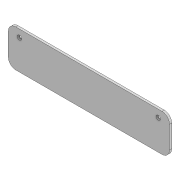
# Autodesk Inventor part: rackback
Saved by Autodesk Inventor 2020 (Build 240168000, 168)
## iProperties
Created: 2021-06-15
Part Number: rackback
Material: Generic
Document SubType Name: Modeling
Designer: Aidan Lee
Density: 1 g/cm^3
Appearance: Default
Author: Aidan Lee
Autodesk Inventor part; units mm, degrees
ref_plane "YZ Plane" through (0, 0, 0) normal (1, 0, 0) x (0, 1, 0)
ref_plane "XZ Plane" through (0, 0, 0) normal (0, 1, 0) x (-1, 0, 0)
ref_plane "XY Plane" through (0, 0, 0) normal (0, 0, 1) x (1, 0, 0)
sketch "Sketch1" plane through (0, 0, 0) normal (0, 0, 1) x (1, 0, 0)
  line L0 (0, 0) -> (215.985, 0)
  line L1 (215.985, 0) -> (215.985, 50)
  line L2 (215.985, 50) -> (0, 50)
  line L3 (0, 50) -> (0, 0)
  circle A0 centre (15, 40) radius 3
  line L4 (107.9925, 95.9564) -> (107.9925, 80.5337) construction
  circle A1 centre (200.985, 40) radius 3
  point P0 (107.9925, 50)
  point P1 (107.9925, 88.2451)
  dimension "d0" = 50
  dimension "d1" = 215.985
  dimension "d2" = 6
  dimension "d3" = 15
  dimension "d4" = 10
  constraints: 10 end point, 2 centre point, 2 midpoint, 2 parallel, 1 horizontal, 1 perpendicular, 1 symmetric about line, 1 vertical, 1 vertical alignment, 1 other
  measures "d0" distance of L2.end L0.start
  measures "d1" distance of L0.start L0.end
  measures "d2" diameter of A0
  measures "d3" distance from line of L3 A0.centre
  measures "d4" distance from line of L2 A0.centre
extrude "Extrusion1" add sketch "Sketch1" along normal blind 3
fillet "Fillet1" radius 10 4 edges at (215.985, 50, 1.5) (0, 50, 1.5) (215.985, 0, 1.5) (0, 0, 1.5)
body "Solid1"
